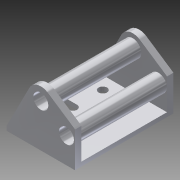
# Autodesk Inventor part: garage door hinge
Saved by Autodesk Inventor 2015 SP1 (Build 190203100, 203)
## iProperties
Created: 2015-01-12
Part Number: garage door hinge
Material: Aluminum 6061
Document SubType Name: Modeling
Designer: Jarod
Density: 2.7 g/cm^3
Appearance: Aluminum - Flat
Author: Jarod
Autodesk Inventor part; units mm, degrees
ref_plane "YZ Plane" through (0, 0, 0) normal (1, 0, 0) x (0, 1, 0)
ref_plane "XZ Plane" through (0, 0, 0) normal (0, 1, 0) x (-1, 0, 0)
ref_plane "XY Plane" through (0, 0, 0) normal (0, 0, 1) x (1, 0, 0)
sketch "Sketch1" plane through (0, 0, 0) normal (0, 1, 0) x (-1, 0, 0)
  line L0 (0, 0) -> (-76.2, 0)
  line L1 (-76.2, 0) -> (-76.2, -63.5) construction
  line L2 (-76.2, -63.5) -> (0, -63.5)
  line L3 (0, -63.5) -> (0, 0) construction
  line L4 (0, -31.75) -> (44.45, -31.75) construction
  line L5 (-76.2, -31.75) -> (-127, -31.75) construction
  circle A0 centre (44.45, -31.75) radius 3.175
  circle A1 centre (-127, -31.75) radius 3.175 construction
  circle A2 centre (-114.3, -31.75) radius 3.175 construction
  line L6 (-114.3, -34.925) -> (-127, -34.925)
  line L7 (-114.3, -28.575) -> (-127, -28.575)
  arc A3 (-114.3, -34.925) -> (-114.3, -28.575) centre (-114.3, -31.75) ccw
  arc A4 (-127, -28.575) -> (-127, -34.925) centre (-127, -31.75) ccw
  line L8 (0, -63.5) -> (47.5152, -37.3112)
  line L9 (47.5152, -26.1888) -> (0, 0)
  line L10 (-76.2, -63.5) -> (-129.7757, -37.4612)
  line L11 (-129.7757, -26.0388) -> (-76.2, 0)
  arc A5 (47.5152, -37.3112) -> (47.5152, -26.1888) centre (44.45, -31.75) ccw
  arc A6 (-129.7757, -26.0388) -> (-129.7757, -37.4612) centre (-127, -31.75) ccw
  circle A7 centre (-76.2, -31.75) radius 3.175 construction
  circle A8 centre (-63.5, -31.75) radius 3.175 construction
  line L12 (-76.2, -28.575) -> (-63.5, -28.575) construction
  line L13 (-76.2, -34.925) -> (-63.5, -34.925) construction
  line L14 (-63.5, -28.575) -> (-76.2, -28.575)
  line L15 (-76.2, -34.925) -> (-63.5, -34.925)
  arc A9 (-63.5, -34.925) -> (-63.5, -28.575) centre (-63.5, -31.75) ccw
  arc A10 (-76.2, -28.575) -> (-76.2, -34.925) centre (-76.2, -31.75) ccw
  circle A11 centre (0, -31.75) radius 3.175 construction
  circle A12 centre (-12.7, -31.75) radius 3.175 construction
  line L16 (0, -28.575) -> (-12.7, -28.575) construction
  line L17 (0, -34.925) -> (-12.7, -34.925) construction
  arc A13 (-12.7, -28.575) -> (-12.7, -34.925) centre (-12.7, -31.75) ccw
  arc A14 (0, -34.925) -> (0, -28.575) centre (0, -31.75) ccw
  line L18 (-12.7, -34.925) -> (0, -34.925)
  line L19 (-12.7, -28.575) -> (0, -28.575)
  dimension "d0" = 76.2
  dimension "d1" = 63.5
  dimension "d2" = 44.45
  dimension "d3" = 50.8
  dimension "d4" = 6.35
  dimension "d5" = 6.35
  dimension "d6" = 6.35
  dimension "d7" = 12.7
  dimension "d8" = 6.35
  dimension "d9" = 0
  dimension "d10" = 0
  dimension "d11" = 0
  dimension "d12" = 0
  dimension "d13" = 6.35
  dimension "d14" = 6.35
  dimension "d15" = 12.7
  dimension "d16" = 0
  dimension "d17" = 6.35
  dimension "d18" = 6.35
  dimension "d19" = 0
  dimension "d20" = 12.7
  constraints: 40 end point, 28 point on circle, 23 tangent, 15 centre point, 5 point on line, 4 coincident, 3 equal length, 3 horizontal, 2 equal radius, 2 midpoint, 1 perpendicular
  measures "d0" distance of L2.end L1.end
  measures "d1" distance of L1.end L0.end
  measures "d2" distance of L4.start L4.end
  measures "d3" distance of L5.start L5.end
  measures "d4" diameter of A0
  measures "d5" diameter of A1
  measures "d6" diameter of A2
  measures "d7" distance of L5.end A2.centre
  measures "d8" radius of A5
  measures "d9" distance of L4.end A5.centre
  measures "d10" distance of L4.end A5.centre
  measures "d11" distance of A4.centre A6.centre
  measures "d12" distance of L5.end A6.centre
  measures "d13" diameter of A7
  measures "d14" diameter of A8
  measures "d15" distance of L5.start A8.centre
  measures "d16" vertical distance of L5.start A8.centre
  measures "d17" diameter of A11
  measures "d18" diameter of A12
  measures "d19" vertical distance of L4.start A12.centre
  measures "d20" distance of L4.start A12.centre
extrude "Extrusion1" add sketch "Sketch1" along normal blind 3.175
sketch "Sketch2" plane through (0, 0, 0) normal (0, 0, 1) x (1, 0, 0)
  line L0 (0, 0) -> (76.2, 0) projected
  line L1 (76.2, 0) -> (76.2, 3.175) projected
  line L2 (0, 3.175) -> (76.2, 3.175) projected
  line L3 (0, 0) -> (0, 3.175) projected
  circle A0 centre (25.4, 31.75) radius 5.5562
  circle A1 centre (44.45, 19.05) radius 5.5563
  line L4 (0, 3.175) -> (16.9289, 36.1049)
  line L5 (30.6835, 39.6753) -> (49.7335, 26.9753)
  line L6 (50.8395, 26.114) -> (76.2, 3.175)
  arc A2 (30.6835, 39.6753) -> (16.9289, 36.1049) centre (25.4, 31.75) ccw
  arc A3 (50.8395, 26.114) -> (49.7335, 26.9753) centre (44.45, 19.05) ccw
  dimension "d23" = 11.1125
  dimension "d24" = 31.75
  dimension "d25" = 25.4
  dimension "d26" = 11.1125
  dimension "d27" = 19.05
  dimension "d28" = 31.75
  dimension "d29" = 9.525
  constraints: 6 end point, 4 centre point, 4 point on circle, 4 tangent, 2 coincident, 1 equal radius
  measures "d23" diameter of A0
  measures "d24" distance from line of L0 A0.centre
  measures "d25" horizontal distance of point (0, 0) A0.centre
  measures "d26" diameter of A1
  measures "d27" distance from line of L0 A1.centre
  measures "d28" distance from line of L1 A1.centre
  measures "d29" radius of A2
extrude "Extrusion2" add sketch "Sketch2" along normal blind 4.7625
sketch "Sketch3" plane through (76.2, 0, -63.5) normal (0, 0, -1) x (-1, 0, 0)
  line L0 (0, 0) -> (76.2, 0) projected
  line L1 (76.2, 0) -> (76.2, 3.175) projected
  line L2 (0, 3.175) -> (76.2, 3.175) projected
  line L3 (0, 0) -> (0, 3.175) projected
  line L4 (59.2711, 36.1049) -> (76.2, 3.175) projected
  arc A0 (59.2711, 36.1049) -> (45.5165, 39.6753) centre (50.8, 31.75) ccw projected
  line L5 (26.4665, 26.9753) -> (45.5165, 39.6753) projected
  arc A1 (26.4665, 26.9753) -> (25.3605, 26.114) centre (31.75, 19.05) ccw projected
  line L6 (0, 3.175) -> (25.3605, 26.114) projected
  circle A2 centre (31.75, 19.05) radius 5.5563 projected
  circle A3 centre (50.8, 31.75) radius 5.5562 projected
  line L7 (76.2, 0) -> (0, 0) projected
  line L8 (0, 0) -> (0, 3.175) projected
  line L9 (76.2, 3.175) -> (76.2, 0) projected
extrude "Extrusion3" add sketch "Sketch3" along normal blind 4.7625
sketch "Sketch5" plane through (0, 0, 0) normal (0, 0, -1) x (-1, 0, 0)
  line L0 (0, 3.175) -> (-76.2, 3.175) projected
  line L1 (-16.9289, 36.1049) -> (0, 3.175) projected
  arc A0 (-16.9289, 36.1049) -> (-30.6835, 39.6753) centre (-25.4, 31.75) ccw projected
  line L2 (-49.7335, 26.9753) -> (-30.6835, 39.6753) projected
  arc A1 (-49.7335, 26.9753) -> (-50.8395, 26.114) centre (-44.45, 19.05) ccw projected
  line L3 (-76.2, 3.175) -> (-50.8395, 26.114) projected
  circle A2 centre (-44.45, 19.05) radius 5.5563 projected
  circle A3 centre (-25.4, 31.75) radius 5.5562 projected
  circle A4 centre (-44.45, 19.05) radius 6.35
  circle A5 centre (-25.4, 31.75) radius 6.35
  point P0 (0, 0)
  dimension "d38" = 12.7
  dimension "d39" = 12.7
  constraints: 2 centre point, 2 coincident
  measures "d38" diameter of A4
  measures "d39" diameter of A5
extrude "Extrusion5" add sketch "Sketch5" along normal blind 63.5 contours A4 | A5
sketch "Sketch6" plane through (0, 3.175, 0) normal (0, 1, 0) x (1, 0, 0)
  line L0 (0, 34.925) -> (12.7, 34.925) projected
  arc A0 (12.7, 28.575) -> (12.7, 34.925) centre (12.7, 31.75) ccw projected
  line L1 (12.7, 28.575) -> (0, 28.575) projected
  arc A1 (0, 34.925) -> (0, 28.575) centre (0, 31.75) ccw projected
  arc A2 (63.5, 34.925) -> (63.5, 28.575) centre (63.5, 31.75) ccw projected
  line L2 (63.5, 34.925) -> (76.2, 34.925) projected
  arc A3 (76.2, 28.575) -> (76.2, 34.925) centre (76.2, 31.75) ccw projected
  line L3 (76.2, 28.575) -> (63.5, 28.575) projected
  arc A4 (127, 28.575) -> (127, 34.925) centre (127, 31.75) ccw projected
  line L4 (127, 28.575) -> (114.3, 28.575) projected
  arc A5 (114.3, 34.925) -> (114.3, 28.575) centre (114.3, 31.75) ccw projected
  line L5 (114.3, 34.925) -> (127, 34.925) projected
  circle A6 centre (-44.45, 31.75) radius 3.175 projected
  line L6 (0, 0) -> (76.2, 0) projected
  line L7 (76.2, 0) -> (129.7757, 26.0388) projected
  arc A7 (129.7757, 26.0388) -> (129.7757, 37.4612) centre (127, 31.75) ccw projected
  line L8 (129.7757, 37.4612) -> (76.2, 63.5) projected
  line L9 (76.2, 63.5) -> (0, 63.5) projected
  line L10 (0, 63.5) -> (-47.5152, 37.3112) projected
  arc A8 (-47.5152, 37.3112) -> (-47.5152, 26.1888) centre (-44.45, 31.75) ccw projected
  line L11 (-47.5152, 26.1888) -> (0, 0) projected
  circle A9 centre (88.9, 31.75) radius 3.175
  circle A10 centre (63.5, 9.525) radius 3.175
  circle A11 centre (63.5, 53.975) radius 3.175
  circle A12 centre (-12.7, 31.75) radius 3.175
  circle A13 centre (12.7, 9.525) radius 3.175
  circle A14 centre (12.7, 53.975) radius 3.175
  dimension "d42" = 6.35
  dimension "d43" = 6.35
  dimension "d44" = 6.35
  dimension "d45" = 6.35
  dimension "d46" = 6.35
  dimension "d47" = 6.35
  dimension "d50" = 22.225
  dimension "d51" = 22.225
  dimension "d52" = 0
  dimension "d53" = 0
  dimension "d54" = 0
  dimension "d55" = 12.7
  dimension "d56" = 12.7
  dimension "d57" = 0
  dimension "d58" = 0
  dimension "d59" = 0
  dimension "d60" = 22.225
  dimension "d61" = 22.225
  constraints: 6 centre point
  measures "d42" diameter of A9
  measures "d43" diameter of A10
  measures "d44" diameter of A11
  measures "d45" diameter of A12
  measures "d46" diameter of A13
  measures "d47" diameter of A14
  measures "d50" distance of A11.centre A2.centre
  measures "d51" distance of A2.centre A10.centre
  measures "d52" horizontal distance of A10.centre A2.centre
  measures "d53" horizontal distance of A11.centre A2.centre
  measures "d54" vertical distance of A9.centre A3.centre
  measures "d55" distance of A3.centre A9.centre
  measures "d56" distance of A1.centre A12.centre
  measures "d57" vertical distance of A12.centre A1.centre
  measures "d58" horizontal distance of A0.centre A13.centre
  measures "d59" horizontal distance of A0.centre A14.centre
  measures "d60" distance of A0.centre A13.centre
  measures "d61" distance of A0.centre A14.centre
extrude "Extrusion6" cut sketch "Sketch6" against normal blind 63.5 contours A9 | A10 | A11 | A12 | A13 | A14
sketch "Sketch7" plane through (0, 0, 0) normal (0, -1, 0) x (1, 0, 0)
  circle A0 centre (12.7, -9.525) radius 3.175 projected
  circle A1 centre (63.5, -53.975) radius 3.175 projected
  circle A2 centre (88.9, -31.75) radius 3.175 projected
  circle A3 centre (63.5, -9.525) radius 3.175 projected
  circle A4 centre (-12.7, -31.75) radius 3.175 projected
  circle A5 centre (12.7, -53.975) radius 3.175 projected
  line L0 (12.7, -34.925) -> (0, -34.925) projected
  arc A6 (0, -28.575) -> (0, -34.925) centre (0, -31.75) ccw projected
  line L1 (0, -28.575) -> (12.7, -28.575) projected
  arc A7 (12.7, -34.925) -> (12.7, -28.575) centre (12.7, -31.75) ccw projected
  arc A8 (63.5, -28.575) -> (63.5, -34.925) centre (63.5, -31.75) ccw projected
  line L2 (63.5, -28.575) -> (76.2, -28.575) projected
  arc A9 (76.2, -34.925) -> (76.2, -28.575) centre (76.2, -31.75) ccw projected
  line L3 (76.2, -34.925) -> (63.5, -34.925) projected
  arc A10 (127, -34.925) -> (127, -28.575) centre (127, -31.75) ccw projected
  line L4 (127, -34.925) -> (114.3, -34.925) projected
  arc A11 (114.3, -28.575) -> (114.3, -34.925) centre (114.3, -31.75) ccw projected
  line L5 (114.3, -28.575) -> (127, -28.575) projected
  circle A12 centre (-44.45, -31.75) radius 3.175 projected
  line L6 (-47.5152, -26.1888) -> (0, 0) projected
  arc A13 (-47.5152, -26.1888) -> (-47.5152, -37.3112) centre (-44.45, -31.75) ccw projected
  line L7 (0, -63.5) -> (-47.5152, -37.3112) projected
  line L8 (129.7757, -37.4612) -> (76.2, -63.5) projected
  arc A14 (129.7757, -37.4612) -> (129.7757, -26.0388) centre (127, -31.75) ccw projected
  line L9 (76.2, 0) -> (129.7757, -26.0388) projected
  line L10 (76.2, 0) -> (76.2, 4.7625) projected
  line L11 (0, 4.7625) -> (76.2, 4.7625) projected
  line L12 (0, 0) -> (0, 4.7625) projected
  line L13 (76.2, 4.7625) -> (50.8, 4.7625) construction
  line L14 (0, 4.7625) -> (76.2, 4.7625) construction
  line L15 (50.8, 4.7625) -> (133.35, 4.7625)
  line L16 (133.35, 4.7625) -> (133.35, -71.4375)
  line L17 (133.35, -71.4375) -> (50.8, -71.4375)
  line L18 (50.8, -71.4375) -> (50.8, 4.7625)
  line L19 (0, -63.5) -> (0, -68.2625) projected
  line L20 (76.2, -68.2625) -> (0, -68.2625) projected
  line L21 (76.2, -63.5) -> (76.2, -68.2625) projected
  dimension "d64" = 25.4
  dimension "d65" = 82.55
  dimension "d66" = 76.2
  constraints: 10 end point, 2 parallel, 1 horizontal, 1 perpendicular, 1 point on line
  measures "d64" distance of L10.end L13.end
  measures "d65" distance of L16.end L17.end
  measures "d66" distance of L15.end L16.end
extrude "Extrusion7" cut sketch "Sketch7" against normal blind 63.5 contours L11 L10 L9 A14 L8 L21 L20 L18 | L15 L16 A14 L9 L10 | L20 L21 L8 A14 L16 L17 L18
sketch "Sketch8" plane through (0, 3.175, 0) normal (0, 1, 0) x (1, 0, 0)
  circle A0 centre (-44.45, 31.75) radius 3.175 projected
  circle A1 centre (-12.7, 31.75) radius 3.175 projected
  line L0 (0, 63.5) -> (-63.5, 63.5)
  line L1 (-63.5, 63.5) -> (-63.5, 0)
  line L2 (-63.5, 0) -> (0, 0)
  line L3 (0, 0) -> (0, 63.5)
  dimension "d69" = 63.5
  dimension "d70" = 63.5
  constraints: 8 end point, 2 parallel, 1 horizontal, 1 perpendicular
  measures "d69" distance of L2.end L1.end
  measures "d70" distance of L1.end L0.end
extrude "Extrusion8" cut sketch "Sketch8" against normal blind 25.4
body "Solid1"
